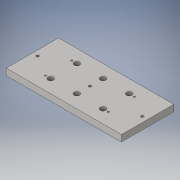
# Autodesk Inventor part: X95carrier-to-M605-adapter-V1
Saved by Autodesk Inventor 2016 (Build 200138000, 138)
## iProperties
Created: 2018-06-26
Part Number: X95carrier-to-M605-adapter-V1
Material: Generic
Document SubType Name: Modeling
Designer: voigt
Density: 1 g/cm^3
Appearance: Default
Author: voigt
Autodesk Inventor part; units mm, degrees
ref_plane "YZ Plane" through (0, 0, 0) normal (1, 0, 0) x (0, 1, 0)
ref_plane "XZ Plane" through (0, 0, 0) normal (0, 1, 0) x (-1, 0, 0)
ref_plane "XY Plane" through (0, 0, 0) normal (0, 0, 1) x (1, 0, 0)
sketch "Sketch1" plane through (0, 0, 0) normal (0, 0, 1) x (1, 0, 0)
  line L0 (0, 70) -> (0, -70) construction
  line L1 (-154, 0) -> (154, 0) construction
  line L2 (-110, 50) -> (110, 50)
  line L3 (110, 50) -> (110, -50)
  line L4 (110, -50) -> (-110, -50)
  line L5 (-110, -50) -> (-110, 50)
  point P0 (0, 0)
  dimension "d0" = 100
  dimension "d1" = 220
  dimension "d2" = 110
  constraints: 8 end point, 2 parallel, 1 horizontal, 1 perpendicular, 1 other
  measures "d0" distance between parallel lines of L4 L2
  measures "d1" distance between parallel lines of L5 L3
  measures "d2" distance between parallel lines of L0 L3
extrude "Extrusion1" add sketch "Sketch1" along normal blind 12.5
sketch "Sketch2" plane through (0, 0, 12.5) normal (0, 0, 1) x (1, 0, 0)
  line L0 (110, 50) -> (-110, 50) construction
  line L1 (-110, 50) -> (-110, -50) construction
  line L2 (-110, -50) -> (110, -50) construction
  line L3 (110, -50) -> (110, 50) construction
  line L4 (-60, 25) -> (60, 25) construction
  line L5 (60, 25) -> (60, -25) construction
  line L6 (60, -25) -> (-60, -25) construction
  line L7 (-60, -25) -> (-60, 25) construction
  line L8 (0, 70) -> (0, -70) construction
  line L9 (-154, 0) -> (154, 0) construction
  point P0 (0, 0)
  dimension "d5" = 50
  dimension "d6" = 120
  constraints: 8 end point, 4 coincident, 2 parallel, 1 horizontal, 1 perpendicular, 2 other
  measures "d5" distance between parallel lines of L6 L4
  measures "d6" distance between parallel lines of L5 L7
hole "Hole1" at (-60, 25, 12.5) at (-60, -25, 12.5) at (60, -25, 12.5) at (60, 25, 12.5) direction (0, 0, -1) diameter 3.242 end through all thread size "M4x0.7" class "6H" standard "ANSI Metric M Profile"
sketch "Sketch3" plane through (0, 0, 12.5) normal (0, 0, 1) x (1, 0, 0)
  circle A0 centre (60, -25) radius 1.621 construction
  circle A1 centre (-60, 25) radius 1.621 construction
  circle A2 centre (-60, -25) radius 1.621 construction
  circle A3 centre (60, 25) radius 1.621 construction
  line L0 (110, 50) -> (-110, 50) construction
  line L1 (-110, 50) -> (-110, -50) construction
  line L2 (-110, -50) -> (110, -50) construction
  line L3 (110, -50) -> (110, 50) construction
  line L4 (0, 70) -> (0, -70) construction
  line L5 (-154, 0) -> (154, 0) construction
  point P0 (0, 0)
  point P1 (-100, 0)
  point P2 (100, 0)
  dimension "d14" = 100
  dimension "d39" = 100
  constraints: 2 point on line
  measures "d14" distance of point (0, 0) point (-100, 0)
  measures "d39" distance from line of L4 point (100, 0)
hole "Hole2" at (-100, 0, 12.5) at (100, 0, 12.5) at (0, 0, 12.5) direction (0, 0, -1) diameter 4.917 end through all thread size "M6x1" class "6H" standard "ANSI Metric M Profile"
sketch "Sketch4" plane through (0, 0, 12.5) normal (0, 0, 1) x (1, 0, 0)
  circle A0 centre (-100, 0) radius 2.4585 construction
  circle A1 centre (60, -25) radius 1.621 construction
  circle A2 centre (-60, 25) radius 1.621 construction
  circle A3 centre (-60, -25) radius 1.621 construction
  circle A4 centre (60, 25) radius 1.621 construction
  line L0 (110, 50) -> (-110, 50) construction
  line L1 (-110, 50) -> (-110, -50) construction
  line L2 (-110, -50) -> (110, -50) construction
  line L3 (110, -50) -> (110, 50) construction
  line L4 (0, 70) -> (0, -70) construction
  line L5 (-154, 0) -> (154, 0) construction
  point P0 (0, 0)
  point P1 (-50, 25)
  point P2 (0, 25)
  point P3 (50, 25)
  point P4 (-50, -25)
  point P5 (0, -25)
  point P6 (50, -25)
  dimension "d22" = 50
  dimension "d23" = 25
  dimension "d26" = 50
  dimension "d29" = 50
  constraints: 1 horizontal, 1 vertical, 5 other
  measures "d22" distance from line of L4 point (-50, 25)
  measures "d23" distance from line of L5 point (-50, 25)
  measures "d26" distance of point (-50, 25) point (0, 25)
  measures "d29" distance of point (-50, 25) point (-50, -25)
hole "Hole3" at (-50, 25, 12.5) at (0, 25, 12.5) at (50, 25, 12.5) at (-50, -25, 12.5) at (0, -25, 12.5) at (50, -25, 12.5) direction (0, 0, -1) diameter 6 end through all counterbore diameter 10.5 counterbore depth 7
body "Solid1"
